Autodesk Inventor part; units mm, degrees
(part 2 of 2)
sketch "Sketch12" plane through (-32, 31.5, 3) normal (0, 1, 0) x (1, 0, 0)
  line L0 (0, 17) -> (0, 0) projected
  line L1 (64, 0) -> (0, 0) projected
  line L2 (64, 0) -> (64, 17) projected
  line L3 (0, 17) -> (64, 17) projected
  line L4 (-10, 17) -> (-7, 17) projected
  line L5 (-10, 0) -> (-10, 17) projected
  line L6 (0, 0) -> (-10, 0) projected
  line L7 (0, 17) -> (0, 0) projected
  line L8 (-2.5, 17) -> (0, 17) projected
  line L9 (-2.5, 3) -> (-2.5, 17) projected
  line L10 (-7, 3) -> (-2.5, 3) projected
  line L11 (-7, 17) -> (-7, 3) projected
  line L12 (64, 17) -> (66.5, 17) projected
  line L13 (64, 0) -> (64, 17) projected
  line L14 (74, 0) -> (64, 0) projected
  line L15 (74, 17) -> (74, 0) projected
  line L16 (71, 17) -> (74, 17) projected
  line L17 (71, 3) -> (71, 17) projected
  line L18 (66.5, 3) -> (71, 3) projected
  line L19 (66.5, 17) -> (66.5, 3) projected
  line L20 (19.7775, 4.6) -> (19.7775, 5.6) projected
  line L21 (32.7725, 4.6) -> (32.7725, 5.6) projected
  line L22 (-2.5, 3) -> (22.5, 3)
  line L23 (22.5, 3) -> (22.5, 17)
  line L24 (22.5, 17) -> (-2.5, 17)
  line L25 (-2.5, 17) -> (-2.5, 3)
  line L26 (66.5, 3) -> (71, 3) projected
  line L27 (66.5, 3) -> (31.5, 3)
  line L28 (31.5, 3) -> (31.5, 17)
  line L29 (31.5, 17) -> (66.5, 17)
  line L30 (66.5, 17) -> (66.5, 3)
  point P0 (32, 3)
  dimension "d87" = 25
  dimension "d88" = 14
  dimension "d89" = 35
  dimension "d90" = 14
  constraints: 16 end point, 4 parallel, 2 horizontal, 2 perpendicular
  measures "d87" distance of L24.end L23.end
  measures "d88" distance of L23.end L22.end
  measures "d89" distance of L28.end L29.end
  measures "d90" distance of L27.end L28.end
extrude "Extrusion11" cut sketch "Sketch12" against normal blind 20 contours L3 L23 L22 L0 | L0 L22 L9 L8 | L3 L2 L27 L28 | L12 L19 L27 L2
sketch "Sketch13" plane through (42, -21.5, 3) normal (1, 0, 0) x (0, 0, -1)
  line L0 (5.6, 39.6525) -> (5.6, 27.2525) projected
  line L1 (5.6, 28.2225) -> (5.6, 15.8225) projected
  line L2 (5.6, 16.7925) -> (5.6, 4.3925) projected
  line L3 (5.6, 37.0225) -> (5.6, 7.0225) construction
  line L4 (3.6, 37.0225) -> (3.6, 7.0225)
  line L5 (7.6, 7.0225) -> (7.6, 37.0225)
  arc A0 (7.6, 37.0225) -> (3.6, 37.0225) centre (5.6, 37.0225) ccw
  arc A1 (3.6, 7.0225) -> (7.6, 7.0225) centre (5.6, 7.0225) ccw
  line L6 (5.6, 22.0225) -> (8.6, 22.0225)
  line L7 (8.6, 37.0225) -> (8.6, 7.0225) construction
  line L8 (6.6, 37.0225) -> (6.6, 7.0225)
  line L9 (10.6, 7.0225) -> (10.6, 37.0225)
  arc A2 (10.6, 37.0225) -> (6.6, 37.0225) centre (8.6, 37.0225) ccw
  arc A3 (6.6, 7.0225) -> (10.6, 7.0225) centre (8.6, 7.0225) ccw
  line L10 (8.6, 39.0225) -> (5.6, 39.0225)
  line L11 (8.6, 5.0225) -> (5.6, 5.0225)
  point P0 (3, 21.5)
  dimension "d93" = 15
  dimension "d94" = 4
  dimension "d95" = 3
  dimension "d96" = 15
  dimension "d97" = 4
  constraints: 22 end point, 12 point on circle, 8 tangent, 4 centre point, 3 midpoint, 2 parallel, 1 horizontal, 1 point on line, 1 vertical
  measures "d93" distance of L6.start L3.end
  measures "d94" diameter of A1
  measures "d95" distance of L6.start L6.end
  measures "d96" distance of L6.end L7.end
  measures "d97" diameter of A3
extrude "Extrusion12" cut sketch "Sketch13" against normal blind 5
sketch "Sketch14" plane through (-34.5, -29, 0) normal (0, 1, 0) x (1, 0, 0)
  line L0 (71.5275, 1.6) -> (71.5275, 2.6) projected
  line L1 (59.1275, 1.6) -> (59.1275, 2.6) projected
  line L2 (76.5, 0.6) -> (59.1275, 0.6)
  line L3 (59.1275, 0.6) -> (59.1275, 7.6)
  line L4 (59.1275, 7.6) -> (76.5, 7.6)
  line L5 (76.5, 7.6) -> (76.5, 0.6)
  line L6 (59.1275, 7.6) -> (76.6916, 7.6)
  line L7 (76.6916, 7.6) -> (76.6916, 14.4539)
  line L8 (76.6916, 14.4539) -> (59.1275, 14.4539)
  line L9 (59.1275, 14.4539) -> (59.1275, 7.6)
  point P0 (34.5, 0)
  point P1 (73.5, 7.6)
  constraints: 16 end point, 4 parallel, 2 horizontal, 2 perpendicular
extrude "Extrusion13" cut sketch "Sketch14" against normal blind 5
sketch "Sketch15" plane through (34.5, -29, -0.6) normal (0, 0, -1) x (-1, 0, 0)
  line L0 (9.8725, -2.5) -> (2.5, -2.5) projected
  line L1 (9.8725, 0) -> (9.8725, -2.5) projected
  line L2 (0, 0) -> (9.8725, 0) projected
  line L3 (2.5, -2.5) -> (0, 0) projected
  point P0 (34.5, 29)
extrude "Extrusion14" cut sketch "Sketch15" against normal up to surface (0.6 mm away)
thicken "Thicken1" operation add thickness 1 both sides no extend neighbours yes toward (-1, 0, 0) faces at (24.6275, -29.8333, -4.6667)
sketch "Sketch16" plane through (-32, -31.5, 3) normal (0, -1, 0) x (1, 0, 0)
  line L0 (35.546, -5.6) -> (17.7025, -5.6) projected
  line L1 (26.6242, -5.6) -> (26.6242, -8.1)
  line L2 (30.6242, -11.1) -> (22.6242, -11.1)
  line L3 (22.6242, -11.1) -> (22.6242, -5.1)
  line L4 (22.6242, -5.1) -> (30.6242, -5.1)
  line L5 (30.6242, -5.1) -> (30.6242, -11.1)
  line L6 (30.6242, -11.1) -> (22.6242, -5.1) construction
  line L7 (22.6242, -11.1) -> (30.6242, -5.1) construction
  point P0 (32, -3)
  dimension "d106" = 2.5
  dimension "d107" = 8
  dimension "d108" = 6
  constraints: 14 end point, 3 midpoint, 2 parallel, 2 perpendicular, 1 vertical
  measures "d106" distance of L1.start L1.end
  measures "d107" distance of L2.start L2.end
  measures "d108" distance of L2.end L3.end
extrude "Extrusion15" cut sketch "Sketch16" against normal blind 5
fillet "Fillet1" radius 1 4 edges at (-1.3758, -30.25, -2.1) (-1.3758, -30.25, -8.1) (-9.3758, -30.25, -8.1) (-9.3758, -30.25, -2.1)
sketch "Sketch17" plane through (42, -21.5, 3) normal (1, 0, 0) x (0, 0, -1)
  line L0 (8.6, 5.0225) -> (5.6, 5.0225) projected
  arc A0 (3.6, 7.0225) -> (5.6, 5.0225) centre (5.6, 7.0225) ccw projected
  line L1 (3.6, 7.0225) -> (3.6, 37.0225) projected
  arc A1 (5.6, 39.0225) -> (3.6, 37.0225) centre (5.6, 37.0225) ccw projected
  line L2 (5.6, 39.0225) -> (8.6, 39.0225) projected
  arc A2 (10.6, 37.0225) -> (8.6, 39.0225) centre (8.6, 37.0225) ccw projected
  line L3 (10.6, 37.0225) -> (10.6, 7.0225) projected
  arc A3 (8.6, 5.0225) -> (10.6, 7.0225) centre (8.6, 7.0225) ccw projected
  line L4 (17, 43) -> (0, 43) projected
  line L5 (0, 0) -> (0, 43) projected
  line L6 (0, 0) -> (17, 0) projected
  line L7 (17, 43) -> (17, 0) projected
  line L8 (17, 43) -> (0, 43) projected
  line L9 (3, 53) -> (3, 46) projected
  line L10 (0, 53) -> (3, 53) projected
  line L11 (0, 43) -> (0, 53) projected
  line L12 (17, 43) -> (0, 43) projected
  line L13 (17, 46) -> (17, 43) projected
  line L14 (3, 46) -> (17, 46) projected
  line L15 (3, -10) -> (3, -3) projected
  line L16 (17, -3) -> (3, -3) projected
  line L17 (17, 0) -> (17, -3) projected
  line L18 (0, 0) -> (17, 0) projected
  line L19 (0, -10) -> (0, 0) projected
  line L20 (3, -10) -> (0, -10) projected
  line L21 (17, -3) -> (17, 46) projected
  line L22 (17, -3) -> (3, -3) projected
  line L23 (17, 46) -> (9.1794, 46)
  line L24 (9.1794, 46) -> (9.1794, -3)
  line L25 (9.1794, -3) -> (17, -3)
  line L26 (17, -3) -> (17, 46)
  point P0 (3, 21.5)
  point P1 (9.1794, 38.9367)
  point P2 (9.1794, 5.1083)
  point P3 (9.1794, -3)
  constraints: 8 end point, 2 parallel, 1 horizontal, 1 perpendicular, 1 point on line
extrude "Extrusion16" cut sketch "Sketch17" against normal blind 5 contours A3 L3 A2 L24 L4 L7 L6 | L6 L17 L16 L24 | L24 L14 L13 L4
fillet "Fillet2" radius 1 2 edges at (40.5, 17.4367, -6.1794) (40.5, -16.3917, -6.1794)
sketch "Sketch18" plane through (-32, 31.5, 3) normal (0, 1, 0) x (1, 0, 0)
  circle A0 centre (27, 14.5) radius 1 projected
  circle A1 centre (2.5, 13.5) radius 1 projected
  point P0 (32, 3)
extrude "Extrusion17" cut sketch "Sketch18" against normal blind 200
fillet "Fillet3" radius 2 3 edges at (-0.5, 30.25, 0) (-9.5, 30.25, 0) (23.6275, -30.25, 0)
sketch "Sketch19" plane through (-32, -31.5, 3) normal (0, -1, 0) x (1, 0, 0)
  circle A0 centre (27, -14.5) radius 1 projected
  circle A1 centre (2.5, -13.5) radius 1 projected
  line L0 (29.6242, -11.1) -> (23.6242, -11.1) projected
  arc A2 (22.6242, -10.1) -> (23.6242, -11.1) centre (23.6242, -10.1) ccw projected
  line L1 (22.6242, -10.1) -> (22.6242, -6.1) projected
  arc A3 (23.6242, -5.1) -> (22.6242, -6.1) centre (23.6242, -6.1) ccw projected
  line L2 (23.6242, -5.1) -> (29.6242, -5.1) projected
  arc A4 (30.6242, -6.1) -> (29.6242, -5.1) centre (29.6242, -6.1) ccw projected
  line L3 (30.6242, -6.1) -> (30.6242, -10.1) projected
  arc A5 (29.6242, -11.1) -> (30.6242, -10.1) centre (29.6242, -10.1) ccw projected
  line L4 (55.6275, -17) -> (55.6275, -5) projected
  arc A6 (57.6275, -3) -> (55.6275, -5) centre (57.6275, -5) ccw projected
  line L5 (57.6275, -3) -> (64, -3) projected
  line L6 (64, -3) -> (64, 0) projected
  line L7 (0, 0) -> (64, 0) projected
  line L8 (0, 0) -> (0, -17) projected
  line L9 (55.6275, -17) -> (0, -17) projected
  line L10 (-2.5, -17) -> (55.6275, -17) projected
  line L11 (55.6275, -17) -> (49.6275, -17)
  line L12 (49.6275, -17) -> (49.6275, -5)
  circle A7 centre (49.6275, -5) radius 1.5
  line L13 (49.6275, -5) -> (49.6275, -12)
  circle A8 centre (49.6275, -12) radius 1.5
  line L14 (49.6275, -12) -> (37.6275, -12)
  line L15 (37.6275, -12) -> (37.6275, -5)
  line L16 (37.6275, -5) -> (49.6275, -5)
  line L17 (49.6275, -5) -> (49.6275, -12)
  circle A9 centre (37.6275, -12) radius 1.5
  circle A10 centre (37.6275, -5) radius 1.5
  line L18 (37.6275, -12) -> (17.6275, -12)
  line L19 (17.6275, -12) -> (17.6275, -5)
  line L20 (17.6275, -5) -> (37.6275, -5)
  line L21 (37.6275, -5) -> (37.6275, -12)
  circle A11 centre (17.6275, -12) radius 1.5
  circle A12 centre (17.6275, -5) radius 1.5
  line L22 (17.6275, -12) -> (7.6275, -12)
  line L23 (7.6275, -12) -> (7.6275, -5)
  line L24 (7.6275, -5) -> (17.6275, -5)
  line L25 (17.6275, -5) -> (17.6275, -12)
  circle A13 centre (7.6275, -12) radius 1.5
  circle A14 centre (7.6275, -5) radius 1.5
  point P0 (32, -3)
  dimension "d118" = 6
  dimension "d119" = 12
  dimension "d120" = 3
  dimension "d121" = 7
  dimension "d122" = 3
  dimension "d123" = 12
  dimension "d124" = 7
  dimension "d125" = 3
  dimension "d126" = 3
  dimension "d127" = 20
  dimension "d128" = 7
  dimension "d129" = 3
  dimension "d130" = 3
  dimension "d131" = 10
  dimension "d132" = 7
  dimension "d133" = 3
  dimension "d134" = 3
  constraints: 30 end point, 8 centre point, 8 coincident, 6 parallel, 4 perpendicular, 3 horizontal, 2 point on line
  measures "d118" distance of L4.start L11.end
  measures "d119" distance of L11.end L12.end
  measures "d120" diameter of A7
  measures "d121" distance of L13.start L13.end
  measures "d122" diameter of A8
  measures "d123" distance of L15.end L16.end
  measures "d124" distance of L14.end L15.end
  measures "d125" diameter of A9
  measures "d126" diameter of A10
  measures "d127" distance of L19.end L20.end
  measures "d128" distance of L18.end L19.end
  measures "d129" diameter of A11
  measures "d130" diameter of A12
  measures "d131" distance of L23.end L24.end
  measures "d132" distance of L22.end L23.end
  measures "d133" diameter of A13
  measures "d134" diameter of A14
extrude "Extrusion18" cut sketch "Sketch19" against normal blind 5 contours A8 L14 L12 | L12 A8 | L14 A8 L12 | A9 L18 L14 | L14 L15 A9 | A7 L16 L12 | L12 L16 A7 | L18 A9 L15 | A10 L20 L15 | L15 L16 A10 | A11 L22 L18 | L18 L19 A11 | L16 L20 A10 | L22 A11 L19 | A12 L19 L20 | L20 L24 A12 | A12 L24 L19 | A13 L23 L22 | L22 L23 A13 | A14 L23 L24 | L24 L23 A14
sketch "Sketch20" plane through (-42, -21.5, -14) normal (-1, 0, 0) x (0, 0, 1)
  line L0 (17, 43) -> (0, 43) projected
  line L1 (0, 0) -> (0, 43) projected
  line L2 (0, 0) -> (17, 0) projected
  line L3 (17, 43) -> (17, 0) projected
  line L4 (0, 0) -> (17, 0) projected
  line L5 (0, 0) -> (17, 43)
  line L6 (17, 43) -> (0, 43) projected
  line L7 (0, 43) -> (17, 0)
  line L8 (8.5, 21.5) -> (4.5, 21.5)
  line L9 (8.5, 21.5) -> (12.5, 21.5)
  circle A0 centre (4.5, 21.5) radius 1.5
  circle A1 centre (12.5, 21.5) radius 1.5
  circle A2 centre (4.5, 29.5) radius 1.5
  circle A3 centre (12.5, 29.5) radius 1.5
  circle A4 centre (4.5, 37.5) radius 1.5
  circle A5 centre (12.5, 37.5) radius 1.5
  circle A6 centre (4.5, 13.5) radius 1.5
  circle A7 centre (12.5, 13.5) radius 1.5
  circle A8 centre (4.5, 21.5) radius 1.5
  circle A9 centre (12.5, 21.5) radius 1.5
  circle A10 centre (4.5, 29.5) radius 1.5
  circle A11 centre (12.5, 29.5) radius 1.5
  circle A12 centre (4.5, 5.5) radius 1.5
  circle A13 centre (12.5, 5.5) radius 1.5
  circle A14 centre (4.5, 13.5) radius 1.5
  circle A15 centre (12.5, 13.5) radius 1.5
  circle A16 centre (4.5, 21.5) radius 1.5
  circle A17 centre (12.5, 21.5) radius 1.5
  point P0 (14, 21.5)
  dimension "d137" = 4
  dimension "d138" = 4
  dimension "d139" = 3
  dimension "d140" = 3
  dimension "d143" = 8
  dimension "d146" = 8
  constraints: 18 centre point, 8 end point, 2 coincident, 2 horizontal, 2 vertical, 32 other
  measures "d137" distance of L8.start L8.end
  measures "d138" distance of L8.start L9.end
  measures "d139" diameter of A0
  measures "d140" diameter of A1
  measures "d143" distance of A0.centre A2.centre
  measures "d146" distance of A0.centre A6.centre
extrude "Extrusion19" cut sketch "Sketch20" against normal blind 5 contours A3 L5 | L5 A3 | A2 L7 | L7 A2 | A7 L7 | L7 A7 | A6 L5 | L5 A6 | A0 | A1 | A4 | A5 | A12 | A13
chamfer "Chamfer2" distance 1 angle 45 4 edges at (0, -31.5, 3) (-42, 0, 3) (0, 31.5, 3) (42, 0, 3)
body "Solid1"
